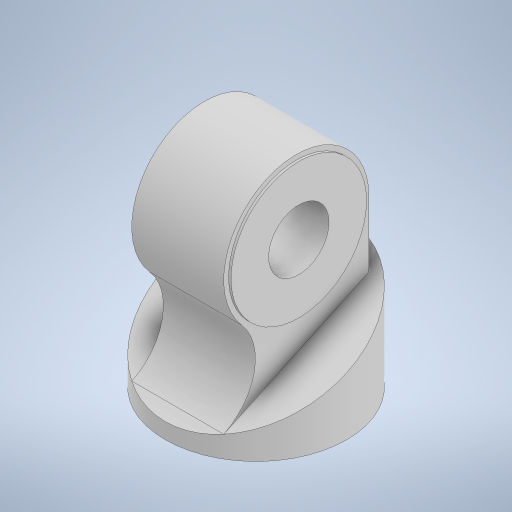
# Autodesk Inventor part: part1
Saved by Autodesk Inventor 2024.1 (Build 281209000, 209)
## iProperties
Created: 2023-08-21
Part Number: part1
Material: Generic
Document SubType Name: Modeling
Designer: admins
Density: 1 g/cm^3
Appearance: Default
Author: admins
Autodesk Inventor part; units mm, degrees
ref_plane "YZ Plane" through (0, 0, 0) normal (1, 0, 0) x (0, 1, 0)
ref_plane "XZ Plane" through (0, 0, 0) normal (0, 1, 0) x (-1, 0, 0)
sketch "Sketch1" plane through (0, 0, 0) normal (0, 1, 0) x (-1, 0, 0)
  circle A0 centre (0, 0) radius 75
  dimension "d0" = 150
  constraints: 1 centre point, 1 coincident
  measures "d0" diameter of A0
extrude "Extrusion1" add sketch "Sketch1" along normal blind 83
ref_plane "Work Plane1" through (71.3599, 83, -75) normal (0, -0.9062, -0.4229) x (1, 0, 0)
sketch "Sketch4" plane through (71.3599, 83, -75) normal (0, -0.9062, -0.4229) x (1, 0, 0)
  line L0 (-176.8472, 196.5702) -> (33.3097, 196.5702)
  line L1 (33.3097, 196.5702) -> (33.3097, -66.4056)
  line L2 (33.3097, -66.4056) -> (-176.8472, -66.4056)
  line L3 (-176.8472, -66.4056) -> (-176.8472, 196.5702)
  point P0 (-71.3599, 103.0632)
  constraints: 8 end point, 2 parallel, 1 horizontal, 1 perpendicular
extrude "Extrusion4" cut sketch "Sketch4" against normal blind 80
sketch "Sketch5" plane through (0, 0, 0) normal (0, -1, 0) x (1, 0, 0)
  circle A0 centre (0, 0) radius 75 projected
  line L0 (38, 64.6607) -> (-38, 64.6607)
  line L1 (-38, 64.6607) -> (-38, -55.3393)
  line L2 (-38, -55.3393) -> (38, -55.3393)
  line L3 (38, -55.3393) -> (38, 64.6607)
  dimension "d9" = 76
  dimension "d10" = 120
  constraints: 8 end point, 2 parallel, 2 point on circle, 1 horizontal, 1 perpendicular
  measures "d9" distance of L2.end L1.end
  measures "d10" distance of L1.end L0.end
extrude "Extrusion5" add sketch "Sketch5" against normal blind 188 contours L3 L2 L1 L0
sketch "Sketch6" plane through (38, 17.825, 64.6607) normal (1, 0, 0) x (0, 0, -1)
  circle A0 centre (60, 110.175) radius 60
  line L0 (0, 170.175) -> (120, 170.175) projected
  line L1 (0, 0) -> (0, 170.175) projected
  circle A1 centre (60, 110.175) radius 56
  line L2 (0, 110.175) -> (0, 0)
  line L3 (0, 0) -> (139.6607, 65.175) projected
  circle A2 centre (-18.8653, 40.855) radius 45
  point P0 (64.6607, -17.825)
  point P1 (0, 110.175)
  point P2 (60, 170.175)
  point P3 (0, 81.7096)
  point P4 (0, 0.0004)
  point P5 (14.9341, 70.5636)
  dimension "d13" = 120
  dimension "d20" = 112
  dimension "d32" = 90
  constraints: 2 centre point, 2 end point, 2 vertical, 1 coincident, 1 collinear, 1 horizontal, 1 point on line, 1 tangent, 4 other
  measures "d20" diameter of A1
  measures "d32" diameter of A2
extrude "Extrusion6" cut sketch "Sketch6" against normal blind 188 contours A0 L1 L0
sketch "Sketch7" plane through (-38, 73.825, -55.3393) normal (-1, 0, 0) x (0, 0, 1)
  circle A0 centre (60, 54.175) radius 60
  line L0 (0, 0) -> (0, 114.175) projected
  line L1 (0, 0) -> (0, 114.175)
  line L2 (60, 114.175) -> (0, 114.175) projected
  line L3 (0, 114.175) -> (60, 114.175)
  line L4 (60, 114.175) -> (0, 114.175)
  circle A1 centre (60, 54.175) radius 56
  circle A2 centre (60, 54.175) radius 25
  point P0 (55.3393, -73.825)
  point P1 (0, 54.175)
  dimension "d16" = 120
  dimension "d23" = 112
  dimension "d26" = 50
  constraints: 6 end point, 2 centre point, 2 coincident, 2 collinear, 2 vertical, 3 other
  measures "d23" diameter of A1
  measures "d26" diameter of A2
extrude "Extrusion7" cut sketch "Sketch7" against normal blind 188 contours A0 L0 L2
extrude "Extrusion8" add sketch "Sketch6" along normal blind 2 contours A1
extrude "Extrusion9" add sketch "Sketch7" along normal blind 2 contours A1 | A2
extrude "Extrusion10" cut sketch "Sketch7" against normal blind 100 contours A2
extrude "Extrusion11" cut sketch "Sketch7" along normal blind 100 contours A2
extrude "Extrusion12" cut sketch "Sketch6" against normal blind 100 contours A2 L1 picked at (2.4551, 28.6667)
extrude "Extrusion13" cut sketch "Sketch6" against normal blind 100 contours A2 L1 A0
body "Solid1"
